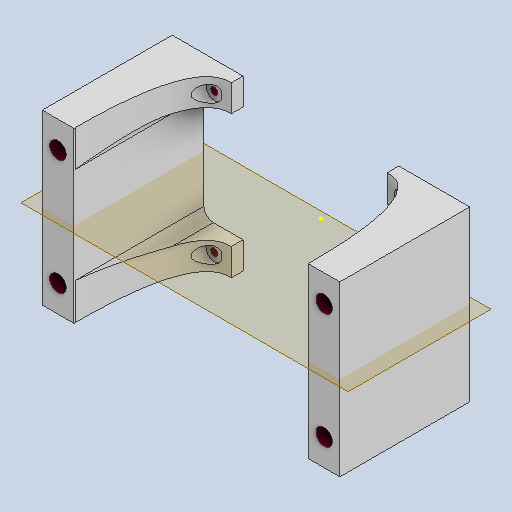
# Autodesk Inventor part: Деталь2
Saved by Autodesk Inventor 2022 (Build 260153000, 153)
## iProperties
Created: 2022-09-15
Part Number: Деталь2
Material: Типовые
Document SubType Name: Modeling
Designer: akapu
Density: 1 g/cm^3
Appearance: По умолчанию
Author: akapu
Autodesk Inventor part; units mm, degrees
ref_plane "YZ Plane" through (0, 0, 0) normal (1, 0, 0) x (0, 1, 0)
ref_plane "XZ Plane" through (0, 0, 0) normal (0, 1, 0) x (-1, 0, 0)
ref_plane "XY Plane" through (0, 0, 0) normal (0, 0, 1) x (1, 0, 0)
sketch "Эскиз1" plane through (0, 0, 0) normal (0, 0, 1) x (1, 0, 0)
  line L0 (-49.6, -20.3) -> (-49.6, 20.4) construction
  line L1 (-17.4076, 24.4) -> (-63.4444, 24.4) construction
  line L2 (-49.6, 0.05) -> (-63.4444, 0.05) construction
  line L3 (-17.4076, -24.3) -> (-63.4444, -24.3) construction
  arc A0 (45.6, -22.3) -> (47.6, -20.3) centre (45.6, -20.3) ccw construction
  line L4 (47.6, -20.3) -> (47.6, 20.4) construction
  arc A1 (47.6, 20.4) -> (45.6, 22.4) centre (45.6, 20.4) ccw construction
  line L5 (45.6, 22.4) -> (-45.6, 22.4) construction
  arc A2 (-45.6, 22.4) -> (-47.6, 20.4) centre (-45.6, 20.4) ccw construction
  line L6 (-47.6, 20.4) -> (-47.6, -20.3) construction
  arc A3 (-47.6, -20.3) -> (-45.6, -22.3) centre (-45.6, -20.3) ccw construction
  line L7 (-45.6, -22.3) -> (45.6, -22.3) construction
  line L8 (-49.6, -20.3) -> (-49.6, 20.4) construction
  arc A4 (-45.6, 24.4) -> (-49.6, 20.4) centre (-45.6, 20.4) ccw construction
  line L9 (-45.6, 24.4) -> (45.6, 24.4) construction
  arc A5 (49.6, 20.4) -> (45.6, 24.4) centre (45.6, 20.4) ccw construction
  line L10 (49.6, 20.4) -> (49.6, -20.3) construction
  arc A6 (45.6, -24.3) -> (49.6, -20.3) centre (45.6, -20.3) ccw construction
  line L11 (45.6, -24.3) -> (-45.6, -24.3) construction
  arc A7 (-49.6, -20.3) -> (-45.6, -24.3) centre (-45.6, -20.3) ccw construction
  arc A8 (-49.6, -20.3) -> (-45.6, -24.3) centre (-45.6, -20.3) ccw
  arc A9 (-45.6, 24.4) -> (-49.6, 20.4) centre (-45.6, 20.4) ccw
  line L12 (-34, 36.75) -> (-62, 36.75) construction
  line L13 (-34, -36.75) -> (-62, -36.75) construction
  line L14 (-63, -85.75) -> (-63, 85.75) construction
  line L15 (-33, -36.75) -> (-33, 36.75)
  line L16 (-33, 36.75) -> (-63, 36.75)
  line L17 (-63, 36.75) -> (-63, -36.75)
  line L18 (-45.6, 24.4) -> (-33, 24.4)
  line L19 (-45.6, -24.3) -> (-33, -24.3)
  line L20 (-63, -36.75) -> (-33, -36.75)
  line L21 (-49.6, 20.4) -> (-49.6, -20.3)
  line L22 (-63, -36.75) -> (-63, -35.75)
  line L23 (-63, -35.75) -> (-33, -35.75)
  line L24 (-63, 36.75) -> (-63, 35.75)
  line L25 (-63, 35.75) -> (-33, 35.75)
  line L26 (-74.5, -92.78) -> (74.5, -92.78) construction
  line L27 (-74.5, -92.78) -> (74.5, -92.78) construction
  line L28 (74.5, 92.75) -> (-74.5, 92.75) construction
  line L29 (0, -92.78) -> (0, 92.75) construction
  line L30 (0, -37.7622) -> (0, 35.75)
  line L31 (63, -85.75) -> (63, 85.75) construction
  line L32 (-63, -35.75) -> (63, -35.75)
  line L33 (-63, 35.75) -> (63, 35.75)
  line L34 (63, -35.75) -> (63, 35.75)
  line L35 (63, 35.75) -> (33, 35.75)
  line L36 (33, 35.75) -> (33, -35.75)
  line L37 (33, -24.3) -> (45.6, -24.3)
  line L38 (49.6, -20.3) -> (49.6, 20.4)
  line L39 (45.6, 24.4) -> (33, 24.4)
  arc A10 (49.6, 20.4) -> (45.6, 24.4) centre (45.6, 20.4) ccw
  arc A11 (45.6, -24.3) -> (49.6, -20.3) centre (45.6, -20.3) ccw
  point P0 (0, 0)
  point P1 (-49.6, 24.4)
  point P2 (49.6, -24.3)
  dimension "d4" = 2
  dimension "d5" = 4
  dimension "d6" = 30
  dimension "d7" = 1
  dimension "d8" = 1
  dimension "d9" = 30
  dimension "d10" = 4
  constraints: 58 end point, 25 point on line, 16 point on circle, 8 centre point, 7 tangent, 6 perpendicular, 3 collinear, 3 midpoint, 2 equal radius, 2 symmetric about line, 1 horizontal, 1 parallel, 7 other
  measures "d4" distance between parallel lines of L9 L5
  measures "d5" radius of A8
  measures "d6" distance of L16.end L15.end
  measures "d7" distance of L17.end L22.end
  measures "d8" distance of L16.end L24.end
  measures "d9" distance of L33.end L35.end
  measures "d10" radius of A10
extrude "Выдавливание1" add sketch "Эскиз1" along normal blind 55 contours A8 L19 L15 L23 L17 L25 L18 A9 L21 | L36 L37 A11 L38 A10 L39 L33 L34 L32
sketch "Эскиз2" plane through (0, 0, 0) normal (0, 0, -1) x (-1, 0, 0)
  circle A0 centre (39.7829, 29.55) radius 1.5 projected
  circle A1 centre (56.3608, 24.4059) radius 1.5 projected
  circle A2 centre (56.3608, -24.4059) radius 1.5 projected
  circle A3 centre (39.7829, -29.55) radius 1.5 projected
  circle A4 centre (-39.7829, -29.55) radius 1.5 projected
  circle A5 centre (-56.3608, -24.4059) radius 1.5 projected
  circle A6 centre (-39.7829, 29.55) radius 1.5 projected
  circle A7 centre (-56.3608, 24.4059) radius 1.5 projected
  point P0 (0, 0)
extrude "Выдавливание2" cut sketch "Эскиз2" against normal through all
sketch "Эскиз4" plane through (-63, -35.75, 0) normal (0, -1, 0) x (1, 0, 0)
  line L0 (0, 55) -> (30, 55) projected
  line L1 (126, 0) -> (126, 55) projected
  line L2 (0, 55) -> (126, 55)
  line L3 (126, 0) -> (96, 0) projected
  line L4 (126, 55) -> (126, 0)
  line L5 (0, 0) -> (30, 0) projected
  line L6 (126, 0) -> (0, 0)
  line L7 (0, 0) -> (0, 55) projected
  line L8 (0, 0) -> (0, 55)
  line L9 (30, 0) -> (30, 55) projected
  line L10 (30, 55) -> (30, 0)
  line L11 (96, 55) -> (108.6, 55) projected
  line L12 (96, 55) -> (96, 0)
  line L13 (63, 55) -> (63, 0)
  line L14 (13.4, 0) -> (13.4, 55) projected
  line L15 (0, 55) -> (13.4, 55)
  line L16 (30, 0) -> (30, 5)
  spline S0 degree 2 poles (13.4, 55) (13.3436, 3.8775) (30, 5) knots 0 0 0 1 1 1
  spline S1 degree 2 poles (112.6, 55) (112.6564, 3.8775) (96, 5) knots 0 0 0 1 1 1
  point P0 (21.1013, 9.5629)
  point P1 (104.8987, 9.5629)
  point P2 (13.4, 54.3127)
  point P3 (96, 5)
  point P4 (112.6, 55)
  dimension "d11" = 5
  constraints: 18 end point, 5 perpendicular, 3 symmetric about line, 2 collinear, 1 midpoint, 1 point on line, 1 vertical, 6 other
  measures "d11" distance of L5.end L16.end
extrude "Выдавливание3" cut sketch "Эскиз4" against normal blind 73 contours L0 L9 S0 | L2 S1 L12
sketch "Эскиз5" plane through (0, 0, 55) normal (0, 0, 1) x (1, 0, 0)
  circle A0 centre (-56.3608, -24.4059) radius 1.5 projected
  circle A1 centre (-56.3608, -24.4059) radius 3.5
  circle A2 centre (-56.3608, 24.4059) radius 1.5 projected
  circle A3 centre (-56.3608, 24.4059) radius 3.5
  circle A4 centre (56.3608, 24.4059) radius 1.5 projected
  circle A5 centre (56.3608, 24.4059) radius 3.5
  circle A6 centre (56.3608, -24.4059) radius 1.5 projected
  circle A7 centre (56.3608, -24.4059) radius 3.5
  point P0 (0, 0)
  dimension "d14" = 7
  dimension "d15" = 7
  dimension "d16" = 7
  dimension "d17" = 7
  constraints: 4 centre point, 4 coincident
  measures "d14" diameter of A1
  measures "d15" diameter of A3
  measures "d16" diameter of A5
  measures "d17" diameter of A7
extrude "Выдавливание4" cut sketch "Эскиз5" against normal blind 45 contours A0 | A1 | A2 | A3 | A4 | A5 | A6 | A7
sketch "Эскиз6" plane through (0, 0, 55) normal (0, 0, 1) x (1, 0, 0)
  circle A0 centre (-39.7829, 29.55) radius 1.5 projected
  circle A1 centre (-39.7829, 29.55) radius 3.5
  circle A2 centre (39.7829, 29.55) radius 1.5 projected
  circle A3 centre (39.7829, 29.55) radius 3.5
  circle A4 centre (39.7829, -29.55) radius 1.5 projected
  circle A5 centre (39.7829, -29.55) radius 3.5
  circle A6 centre (-39.7829, -29.55) radius 1.5 projected
  circle A7 centre (-39.7829, -29.55) radius 3.5
  point P0 (0, 0)
  dimension "d20" = 7
  dimension "d21" = 7
  dimension "d22" = 7
  dimension "d23" = 7
  constraints: 4 centre point, 4 coincident
  measures "d20" diameter of A1
  measures "d21" diameter of A3
  measures "d22" diameter of A5
  measures "d23" diameter of A7
extrude "Выдавливание5" cut sketch "Эскиз6" against normal blind 49.6 contours A0 | A1 | A2 | A3 | A4 | A5 | A6 | A7
ref_plane "РабПлоскость2" through (33, 0, 0) normal (0, 1, 0) x (1, 0, 0)
sketch "Эскиз7" plane through (33, 0, 0) normal (0, 1, 0) x (1, 0, 0)
  point P0 (-33, 0)
